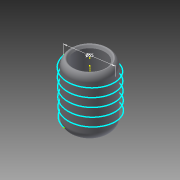
# Autodesk Inventor part: solenoid_looking_pot
Saved by Autodesk Inventor 2015 SP1 (Build 190203100, 203)
## iProperties
Created: 2014-10-09
Part Number: solenoid_looking_pot
Material: Generic
Document SubType Name: Modeling
Designer: dorislee
Density: 1 g/cm^3
Appearance: Default
Author: dorislee
Autodesk Inventor part; units mm, degrees
ref_plane "YZ Plane" through (0, 0, 0) normal (1, 0, 0) x (0, 1, 0)
ref_plane "XZ Plane" through (0, 0, 0) normal (0, 1, 0) x (-1, 0, 0)
ref_plane "XY Plane" through (0, 0, 0) normal (0, 0, 1) x (1, 0, 0)
sketch "Sketch1" plane through (0, 0, 0) normal (0, 0, 1) x (1, 0, 0)
  circle A0 centre (0, 0) radius 25
  dimension "d0" = 50
  constraints: 1 centre point, 1 coincident
  measures "d0" diameter of A0
extrude "Extrusion1" add sketch "Sketch1" along normal blind 70
hole "Hole1" at (0, 0, 70) direction (0, 0, -1) diameter 36 depth 60 tip angle 118 countersink diameter 40 countersink angle 70
fillet "Fillet1" radius 2 1 edges at (0, 20, 70)
sketch "Sketch2" plane through (0, 0, 70) normal (0, 0, 1) x (1, 0, 0)
  point P0 (0, 0)
fillet "Fillet2" radius 10 1 edges at (-25, 0, 0)
fillet "Fillet3" radius 10 1 edges at (-25, 0, 70)
sketch3d "3D Sketch2"
body "Solid1"
